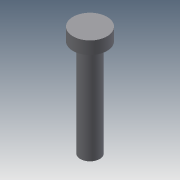
# Autodesk Inventor part: ScrewM2L10
Saved by Autodesk Inventor 2015 SP1 (Build 190203100, 203)
## iProperties
Created: 2015-02-23
Part Number: ScrewM2L10
Material: 一般
Document SubType Name: Modeling
Designer: Yamaura
Density: 1 g/cm^3
Appearance: 既定
Author: Yamaura
Autodesk Inventor part; units mm, degrees
ref_plane "YZ Plane" through (0, 0, 0) normal (1, 0, 0) x (0, 1, 0)
ref_plane "XZ Plane" through (0, 0, 0) normal (0, 1, 0) x (-1, 0, 0)
ref_plane "XY Plane" through (0, 0, 0) normal (0, 0, 1) x (1, 0, 0)
sketch "スケッチ1" plane through (0, 0, 0) normal (1, 0, 0) x (0, 1, 0)
  point P0 (0, 0)
sketch "スケッチ2" plane through (0, 0, 0) normal (1, 0, 0) x (0, 1, 0)
  line L0 (0, 1.3) -> (1.75, 1.3)
  line L1 (1.75, 1.3) -> (1.75, 0)
  line L2 (1.75, 0) -> (1, 0)
  line L3 (1, 0) -> (1, -12)
  line L4 (1, -12) -> (0, -12)
  line L5 (0, 1.3) -> (0, -12)
  point P0 (0, 0)
  dimension "d0" = 1.3
  dimension "d1" = 12
  dimension "d2" = 1
  dimension "d3" = 1.75
  constraints: 12 end point, 4 perpendicular, 2 point on line, 1 vertical
  measures "d0" distance of L0.end L1.end
  measures "d1" distance of L2.end L3.end
  measures "d2" distance of L3.end L4.end
  measures "d3" distance of L0.start L0.end
revolve "回転1" add sketch "スケッチ2" angle 360 about axis through (0, 0, 1.3) along (0, 0, -1)
move faces "移動1" translate (0, 0, 2) faces at (0.3117, 0.1182, -12)
